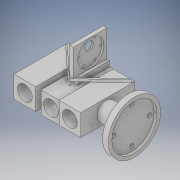
# Autodesk Inventor part: fingers1
Saved by Autodesk Inventor 2018 (Build 220112000, 112)
## iProperties
Created: 2020-03-06
Part Number: fingers1
Material: Generic
Document SubType Name: Modeling
Designer: Jesse R-B
Density: 1 g/cm^3
Appearance: Default
Author: Jesse R-B
Autodesk Inventor part; units mm, degrees
sketch "Sketch1" plane through (0, 0, 0) normal (1, 0, 0) x (0, 1, 0)
  circle A0 centre (0, 0) radius 2.9972
  dimension "d0" = 5.9944
  constraints: 1 centre point, 1 coincident
  measures "d0" diameter of A0
extrude "Extrusion1" add sketch "Sketch1" along normal blind 34.8234
sketch "Sketch2" plane through (34.8234, 0, 0) normal (1, 0, 0) x (0, 0, -1)
  circle A0 centre (0, 0) radius 15.24
  dimension "d3" = 30.48
  constraints: 1 centre point, 1 coincident
  measures "d3" diameter of A0
extrude "Extrusion2" add sketch "Sketch2" against normal blind 12.7
ref_plane "Work Plane1" through (0, 0, 0) normal (0, -0.8660254, 0.5) x (1, 0, 0)
sketch "Sketch7" plane through (0, 0, 0) normal (0, -0.8660254, 0.5) x (1, 0, 0)
  line L0 (34.8234, -9.1805) -> (22.1234, -9.1805) projected
  line L1 (22.1234, 6.4681) -> (22.1234, 5.3565) projected
  line L2 (34.8234, 6.4681) -> (22.1234, 6.4681) projected
  line L3 (34.8234, 6.4681) -> (34.8234, 5.3565) projected
  line L4 (22.1234, 4.8046) -> (34.8234, 4.8046)
  line L5 (34.8234, 4.8046) -> (34.8234, -7.8954)
  line L6 (34.8234, -7.8954) -> (22.1234, -7.8954)
  line L7 (22.1234, -7.8954) -> (22.1234, 4.8046)
  line L8 (22.1234, 2.9972) -> (22.1234, -2.9972) projected
  line L9 (0, 2.9972) -> (0, -2.9972) projected
  line L10 (0, 2.9972) -> (22.1234, 2.9972) projected
  line L11 (22.1234, 5.3565) -> (34.8234, 5.3565) projected
  point P0 (0, 0)
  dimension "d20" = 12.7
  constraints: 8 end point, 2 parallel, 1 horizontal, 1 perpendicular
  measures "d20" distance between parallel lines of L7 L5
extrude "Extrusion5" add sketch "Sketch7" along normal blind 38.1 contours L4 L5 L6 L7
sketch "Sketch8" plane through (34.8234, 0, 0) normal (1, 0, 0) x (0, 0, -1)
  line L0 (-11.3923, -10.1229) -> (-23.2109, -30.5933) projected
  line L1 (-23.2109, -30.5933) -> (-8.5462, -30.5933)
  line L2 (0.3199, -15.2366) -> (-12.2124, -36.9433) projected
  line L3 (-8.5462, -30.5933) -> (-12.2124, -36.9433)
  line L4 (-12.2124, -36.9433) -> (-23.2109, -30.5933)
  point P0 (0, 0)
  point P1 (0.1491, -15.5326)
  point P2 (-0.4582, -16.5843)
  point P3 (-11.957, -11.101)
  point P4 (0.2017, -15.4414)
  point P5 (-11.819, -10.8618)
  constraints: 6 end point, 1 collinear, 1 horizontal, 1 perpendicular, 1 point on line
extrude "Extrusion6" cut sketch "Sketch8" against normal blind 25.4
sketch "Sketch10" plane through (34.8234, -30.5933, 8.5462) normal (0, -1, 0) x (1, 0, 0)
  line L0 (-12.7, 0) -> (-12.7, 14.6647) projected
  line L1 (0, 0) -> (-12.7, 0) projected
  line L2 (0, 14.6647) -> (0, 0) projected
  line L3 (0, 14.6647) -> (-12.7, 14.6647) projected
  point P0 (-34.8234, -8.5462)
sketch "Sketch11" plane through (34.8234, -30.5933, 8.5462) normal (0, -1, 0) x (1, 0, 0)
  line L0 (7.62, 45.4323) -> (-20.32, 45.4323)
  line L1 (-20.32, 45.4323) -> (-20.32, -30.7677)
  line L2 (-20.32, -30.7677) -> (7.62, -30.7677)
  line L3 (7.62, -30.7677) -> (7.62, 45.4323)
  line L4 (0, 14.6647) -> (-12.7, 14.6647) construction
  line L5 (-6.35, 14.6647) -> (-6.35, 45.4323) construction
  line L6 (0, 0) -> (-12.7, 0) construction
  line L7 (-6.35, 0) -> (-6.35, -30.7677) construction
  line L8 (0, 2.8461) -> (0, 14.6647) construction
  line L9 (0, 8.9687) -> (7.62, 8.9687) construction
  line L10 (-12.7, 2.8461) -> (-12.7, 14.6647) construction
  line L11 (-12.7, 8.9687) -> (-20.32, 8.9687) construction
  point P0 (-34.8234, -8.5462)
  point P1 (0, 3.4108)
  point P2 (-12.7, 3.4108)
  point P3 (0, 3.2728)
  point P4 (-12.7, 3.2728)
  dimension "d29" = 27.94
  dimension "d30" = 76.2
  constraints: 16 end point, 6 point on line, 4 midpoint, 3 perpendicular, 2 collinear, 2 parallel, 1 horizontal
  measures "d29" distance between parallel lines of L3 L1
  measures "d30" distance of L2.end L0.start
extrude "Extrusion8" add sketch "Sketch11" along normal blind 30.48
sketch "Sketch13" plane through (14.5034, -30.5933, -22.2214) normal (-1, 0, 0) x (0, 0, 1)
  line L0 (45.6572, -16.7321) -> (32.9572, -16.7321)
  line L1 (32.9572, -16.7321) -> (32.9572, -4.0321)
  line L2 (32.9572, -4.0321) -> (45.6572, -4.0321)
  line L3 (45.6572, -4.0321) -> (45.6572, -16.7321)
  point P0 (22.2214, 30.5933)
  dimension "d37" = 12.7
  dimension "d38" = 12.7
  constraints: 8 end point, 2 parallel, 1 horizontal, 1 perpendicular
  measures "d37" distance of L0.start L0.end
  measures "d38" distance of L0.end L1.end
extrude "Extrusion9" add sketch "Sketch13" along normal blind 2.54
sketch "Sketch14" plane through (11.9634, -30.5933, -22.2214) normal (-1, 0, 0) x (0, 0, 1)
  line L0 (81.28, -25.4) -> (5.08, -25.4)
  line L1 (5.08, -25.4) -> (5.08, 5.08)
  line L2 (5.08, 5.08) -> (81.28, 5.08)
  line L3 (81.28, 5.08) -> (81.28, -25.4)
  line L4 (76.2, 0) -> (0, 0) projected
  line L5 (76.2, 0) -> (76.2, -30.48) projected
  point P0 (22.2214, 30.5933)
  dimension "d41" = 30.48
  dimension "d45" = 76.2
  dimension "d46" = 5.08
  dimension "d47" = 5.08
  constraints: 8 end point, 2 parallel, 1 horizontal, 1 perpendicular
  measures "d41" distance of L2.end L0.start
  measures "d45" distance of L1.end L2.end
  measures "d46" distance between parallel lines of L4 L2
  measures "d47" distance between parallel lines of L5 L3
extrude "Extrusion10" add sketch "Sketch14" along normal blind 30.48
ref_plane "Work Plane2" through (28.4734, -30.5933, -22.2214) normal (-1, 0, 0) x (0, 0, 1)
mirror "Mirror1" about plane through (28.4734, -30.5933, -22.2214) normal (-1, 0, 0) of "Extrusion10", "Extrusion9"
sketch "Sketch15" plane through (11.9634, -55.9933, -17.1414) normal (0, -1, 0) x (1, 0, 0)
  line L0 (33.02, 76.2) -> (33.02, 0) construction
  line L1 (33.02, 0) -> (63.5, 0) construction
  line L2 (63.5, 0) -> (63.5, 76.2) construction
  line L3 (33.02, 76.2) -> (63.5, 76.2) construction
  line L4 (30.48, 71.12) -> (2.54, 71.12) construction
  line L5 (2.54, 71.12) -> (2.54, -5.08) construction
  line L6 (2.54, -5.08) -> (30.48, -5.08) construction
  line L7 (30.48, -5.08) -> (30.48, 71.12) construction
  line L8 (0, 76.2) -> (0, 0) construction
  line L9 (0, 76.2) -> (-30.48, 76.2) construction
  line L10 (-30.48, 0) -> (-30.48, 76.2) construction
  line L11 (0, 0) -> (-30.48, 0) construction
  line L12 (33.02, 0) -> (63.5, 0) construction
  line L13 (63.5, 0) -> (16.7235, 43.4086) construction
  line L14 (0, 0) -> (-30.48, 0) construction
  line L15 (16.7235, 43.4086) -> (-30.48, 0) construction
  circle A0 centre (60.7629, 2.54) radius 2.54 construction
  line L16 (62.4907, 4.4018) -> (18.4513, 45.2705)
  line L17 (59.0352, 0.6782) -> (14.9957, 41.5468)
  arc A1 (59.0352, 0.6782) -> (62.4907, 4.4018) centre (60.7629, 2.54) ccw
  arc A2 (18.4513, 45.2705) -> (14.9957, 41.5468) centre (16.7235, 43.4086) ccw
  point P0 (-11.9634, 17.1414)
  dimension "d50" = 5.08
  dimension "d52" = 5.08
  constraints: 8 end point, 6 point on circle, 3 centre point, 3 tangent, 1 coincident, 1 concentric, 1 parallel, 1 point on line
  measures "d50" diameter of A0
  measures "d52" diameter of A2
extrude "Extrusion11" add sketch "Sketch15" along normal blind 2.54 draft -30
mirror "Mirror2" about plane through (28.4734, -30.5933, -22.2214) normal (-1, 0, 0) of "Extrusion11"
sketch "Sketch16" plane through (14.5034, -30.5933, 53.9786) normal (0, 0, 1) x (1, 0, 0)
  line L0 (27.94, 0) -> (0, 0) projected
  line L1 (0, 0) -> (0, -30.48) projected
  line L2 (27.94, -30.48) -> (0, -30.48) projected
  line L3 (27.94, 0) -> (27.94, -30.48) projected
  circle A0 centre (13.97, -15.24) radius 10.541
  line L4 (30.48, 5.08) -> (30.48, -25.4) projected
  line L5 (30.48, -25.4) -> (60.96, -25.4) projected
  line L6 (60.96, -25.4) -> (60.96, 5.08) projected
  line L7 (30.48, 5.08) -> (60.96, 5.08) projected
  line L8 (-2.54, 5.08) -> (-2.54, -25.4) projected
  line L9 (-2.54, 5.08) -> (-33.02, 5.08) projected
  line L10 (-33.02, -25.4) -> (-33.02, 5.08) projected
  line L11 (-2.54, -25.4) -> (-33.02, -25.4) projected
  circle A1 centre (45.72, -10.16) radius 10.541
  circle A2 centre (-17.78, -10.16) radius 10.541
  point P0 (-14.5034, 30.5933)
  dimension "d56" = 21.082
  dimension "d57" = 21.082
  dimension "d58" = 15.24
  dimension "d59" = 15.24
  dimension "d62" = 15.24
  dimension "d63" = 15.24
  dimension "d64" = 21.082
  dimension "d66" = 13.97
  dimension "d67" = 15.24
  constraints: 3 centre point
  measures "d56" diameter of A1
  measures "d57" diameter of A2
  measures "d58" distance from line of L5 A1.centre
  measures "d59" distance from line of L6 A1.centre
  measures "d62" distance from line of L11 A2.centre
  measures "d63" distance from line of L10 A2.centre
  measures "d64" diameter of A0
  measures "d66" distance from line of L3 A0.centre
  measures "d67" distance from line of L2 A0.centre
extrude "Extrusion12" cut sketch "Sketch16" along normal through all both and the other way through all contours A0 | A1 | A2
ref_plane "Work Plane3" through (-18.5166, -40.7533, 59.0586) normal (0, -1, 0) x (1, 0, 0)
mirror "Mirror3" about plane through (-18.5166, -40.7533, 59.0586) normal (0, -1, 0) of "Extrusion11", "Mirror2"
sketch "Sketch17" plane through (31.4068, -25.5133, 20.278) normal (0, -1, 0) x (1, 0, 0)
  line L0 (-46.456, -35.6663) -> (-2.9334, 4.7228) projected
  arc A0 (-47.9165, -34.0925) -> (-46.456, -35.6663) centre (-47.1863, -34.8794) ccw projected
  line L1 (-3.8771, 6.7761) -> (-47.9165, -34.0925) projected
  arc A1 (-2.9334, 7.0413) -> (-3.8771, 6.7761) centre (-3.1468, 5.9892) ccw projected
  arc A2 (-1.9896, 6.7761) -> (-2.9334, 7.0413) centre (-2.7199, 5.9892) ccw projected
  line L2 (-1.9896, 6.7761) -> (42.0498, -34.0925) projected
  arc A3 (40.5893, -35.6663) -> (42.0498, -34.0925) centre (41.3196, -34.8794) ccw projected
  line L3 (40.5893, -35.6663) -> (-2.9334, 4.7228) projected
  line L4 (-2.9334, 7.0413) -> (-2.9334, 8.5202) projected
  arc A4 (-2.9334, 7.0413) -> (-3.8771, 6.7761) centre (-3.1468, 5.9892) ccw projected
  line L5 (-4.8746, 7.8511) -> (-3.8771, 6.7761) projected
  arc A5 (-2.9334, 8.5202) -> (-4.8746, 7.8511) centre (-3.1468, 5.9892) ccw projected
  line L6 (-2.9334, 7.0413) -> (-2.9334, 8.5202) projected
  arc A6 (-0.9921, 7.8511) -> (-2.9334, 8.5202) centre (-2.7199, 5.9892) ccw projected
  line L7 (-0.9921, 7.8511) -> (-1.9896, 6.7761) projected
  arc A7 (-1.9896, 6.7761) -> (-2.9334, 7.0413) centre (-2.7199, 5.9892) ccw projected
  circle A8 centre (-2.9334, 7.0413) radius 1.4789
  point P0 (-31.4068, -20.278)
  constraints: 1 coincident, 1 vertical alignment, 2 other
extrude "Extrusion13" add sketch "Sketch17" along normal blind 7.62 contours A8 L5 L1 | L1 A1 A2 L2 A8 | L5 A8 L4 A1 | L2 L7 A8 | L4 A8 L7 A2
ref_plane "Work Plane4" through (15.7734, 0, 0) normal (-1, 0, 0) x (0, 0, 1)
sketch "Sketch19" plane through (34.8234, 0, 0) normal (1, 0, 0) x (0, 0, -1)
  line L0 (-27.0541, -22.9733) -> (13.8145, -22.9733) projected
  line L1 (-49.0455, 45.2859) -> (19.1397, 45.2859)
  line L2 (19.1397, 45.2859) -> (19.1397, -22.9733)
  line L3 (19.1397, -22.9733) -> (-49.0455, -22.9733)
  line L4 (-49.0455, -22.9733) -> (-49.0455, 45.2859)
  point P0 (0, 0)
  constraints: 8 end point, 2 parallel, 1 horizontal, 1 perpendicular
extrude "Extrusion15" cut sketch "Sketch19" against normal blind 76.2
sketch "Sketch20" plane through (34.8234, -22.9733, 18.8115) normal (0, 1, 0) x (1, 0, 0)
  line L0 (-12.7, 14.6647) -> (0, 14.6647) projected
  line L1 (-12.7, 0) -> (-12.7, 14.6647) projected
  line L2 (0, 0) -> (-12.7, 0) projected
  line L3 (0, 14.6647) -> (0, 0) projected
  line L4 (39.6307, 31.5511) -> (10.16, 4.2023) projected
  line L5 (10.16, 4.2023) -> (10.16, -40.2471) projected
  line L6 (10.16, -40.2471) -> (40.64, -40.2471) projected
  line L7 (40.64, -40.2471) -> (40.64, 35.9529) projected
  line L8 (37.9029, 35.9529) -> (40.64, 35.9529) projected
  arc A0 (39.6307, 31.5511) -> (37.9029, 35.9529) centre (37.9029, 33.4129) ccw projected
  arc A1 (-50.6029, 35.9529) -> (-52.3307, 31.5511) centre (-50.6029, 33.4129) ccw projected
  line L9 (-50.6029, 35.9529) -> (-53.34, 35.9529) projected
  line L10 (-53.34, -40.2471) -> (-53.34, 35.9529) projected
  line L11 (-22.86, -40.2471) -> (-53.34, -40.2471) projected
  line L12 (-22.86, 4.2023) -> (-22.86, -40.2471) projected
  line L13 (-22.86, 4.2023) -> (-52.3307, 31.5511) projected
  line L14 (-12.7, 0) -> (-12.7, 14.6647) projected
  line L15 (-12.7, 7.3323) -> (0, 7.3323)
  line L16 (0, 7.3323) -> (0, 39.0823)
  line L17 (0, 39.0823) -> (-12.7, 39.0823)
  line L18 (-12.7, 39.0823) -> (-12.7, 7.3323)
  point P0 (-34.8234, 18.8115)
  dimension "d78" = 31.75
  dimension "d79" = 0
  constraints: 8 end point, 2 parallel, 1 horizontal, 1 midpoint, 1 perpendicular
  measures "d78" distance of L17.end L15.start
  measures "d79" distance between parallel lines of L3 L16
extrude "Extrusion16" add sketch "Sketch20" against normal up to surface (7.62 mm away) contours L18 L17 L16 L0 | L0 L3 L15 L1 | L15 L3 L2 L1
ref_plane "Work Plane5" through (28.4734, 0, 0) normal (1, 0, 0) x (0, 0, -1)
sketch "Sketch21" plane through (28.4734, 0, 0) normal (1, 0, 0) x (0, 0, -1)
  circle A0 centre (-0.349, 3.0767) radius 5.9944
  circle A1 centre (15.151, -3.9233) radius 1.4986
  circle A2 centre (7.401, 9.5001) radius 1.4986
  circle A3 centre (-8.099, 9.5001) radius 1.4986
  circle A4 centre (-15.849, -3.9233) radius 1.4986
  circle A5 centre (-8.099, -17.3467) radius 1.4986
  circle A6 centre (7.401, -17.3467) radius 1.4986
  circle A7 centre (-0.349, -3.9233) radius 18.4023
  circle A8 centre (-0.349, -3.9233) radius 18.4023
  line L0 (18.193, 15.1267) -> (15.3215, 15.1267)
  line L1 (-16.0195, 15.1267) -> (15.3215, 15.1267)
  line L2 (-16.0195, 15.1267) -> (-18.891, 15.1267)
  line L3 (-18.891, 15.1267) -> (-18.891, -22.9733)
  line L4 (-16.0195, -22.9733) -> (-18.891, -22.9733)
  line L5 (15.3215, -22.9733) -> (-16.0195, -22.9733)
  line L6 (18.193, -22.9733) -> (15.3215, -22.9733)
  line L7 (18.193, 15.1267) -> (18.193, -22.9733)
  line L8 (-16.0195, 15.1267) -> (15.3215, 15.1267)
  line L9 (-27.0541, -22.9733) -> (13.8145, -22.9733) projected
  line L10 (20.2708, -22.9733) -> (20.2708, -30.5933) projected
  point P0 (0, 0)
  dimension "d82" = 36.8046
  dimension "d83" = 11.9888
  dimension "d84" = 2.9972
  dimension "d85" = 2.9972
  dimension "d86" = 2.9972
  dimension "d87" = 2.9972
  dimension "d88" = 2.9972
  dimension "d89" = 2.9972
  dimension "d90" = 90
  dimension "d91" = 2.8715
  dimension "d92" = 31.341
  dimension "d93" = 31.341
  dimension "d94" = 38.1
  dimension "d95" = 37.084
  dimension "d96" = 7
  dimension "d97" = 18.542
  dimension "d98" = 18.542
  dimension "d99" = 7
  dimension "d100" = 19.05
  dimension "d101" = 6.4234
  dimension "d102" = 7.75
  dimension "d103" = 6.4234
  dimension "d104" = 7.75
  dimension "d105" = 15.5
  dimension "d106" = 9.5144
  dimension "d107" = 15.5
  dimension "d108" = 7
  dimension "d109" = 13.4234
  dimension "d110" = 7.75
  dimension "d111" = 7.75
  dimension "d112" = 20.4234
  dimension "d113" = 0
  dimension "d114" = 2.0778
  dimension "d115" = 15.1267
  constraints: 18 end point, 9 centre point, 2 collinear, 2 concentric
  measures "d82" diameter of A7
  measures "d83" diameter of A0
  measures "d84" diameter of A3
  measures "d85" diameter of A2
  measures "d86" diameter of A1
  measures "d87" diameter of A6
  measures "d88" diameter of A5
  measures "d89" diameter of A4
  measures "d90" angle of L1 L3
  measures "d91" distance from line of L7 L1.end
  measures "d92" distance of L1.start L1.end
  measures "d93" distance of L5.start L4.start
  measures "d94" distance of L0.start L7.end
  measures "d95" distance between parallel lines of L3 L7
  measures "d96" distance of A8.centre A0.centre
  measures "d97" distance from line of L7 A8.centre
  measures "d98" distance from line of L3 A0.centre
  measures "d99" distance of A7.centre A0.centre
  measures "d100" distance from line of A8.centre L5
  measures "d101" vertical distance of A0.centre A2.centre
  measures "d102" horizontal distance of A0.centre A2.centre
  measures "d103" vertical distance of A3.centre A0.centre
  measures "d104" horizontal distance of A3.centre A0.centre
  measures "d105" horizontal distance of A0.centre A4.centre
  measures "d107" horizontal distance of A0.centre A1.centre
  measures "d108" vertical distance of A0.centre A1.centre
  measures "d109" vertical distance of A6.centre A1.centre
  measures "d110" horizontal distance of A1.centre A6.centre
  measures "d111" horizontal distance of A0.centre A5.centre
  measures "d112" vertical distance of A0.centre A5.centre
  measures "d113" distance between parallel lines of L9 L5
  measures "d114" distance between parallel lines of L10 L7
  measures "d115" distance from line of point (0, 0) L1
extrude "Extrusion17" add sketch "Sketch21" along normal mid plane 5.08 contours L7 L6 L5 L4 L3 L2 L1 L0
extrude "Extrusion18" add sketch "Sketch21" against normal blind 2.54 contours A7
sketch "Sketch22" plane through (34.8234, -22.9733, -20.2708) normal (0, 0, -1) x (-1, 0, 0)
  line L0 (6.35, 0.6477) -> (6.35, 37.4523) projected
  line L1 (8.89, 38.1) -> (3.81, 38.1) projected
  line L2 (3.81, 0) -> (3.81, 38.1) projected
  line L3 (8.89, 0) -> (3.81, 0) projected
  line L4 (8.89, 38.1) -> (8.89, 0) projected
  line L5 (12.7, -7.62) -> (0, -7.62) projected
  line L6 (12.7, 0) -> (12.7, -7.62) projected
  line L7 (0, 0) -> (12.7, 0) projected
  line L8 (0, 0) -> (0, -7.62) projected
  point P0 (34.8234, 22.9733)
extrude "Extrusion19" add sketch "Sketch22" against normal up to surface (2.0778 mm away) contours L4 L3 L2 L1
sketch "Sketch23" plane through (34.8234, -30.5933, -20.2708) normal (0, 0, -1) x (-1, 0, 0)
  line L0 (12.7, 0) -> (0, 0) projected
  line L1 (12.7, 7.62) -> (12.7, 0) projected
  line L2 (8.89, 7.62) -> (12.7, 7.62) projected
  line L3 (8.89, 7.62) -> (8.89, 45.72) projected
  line L4 (8.89, 45.72) -> (3.81, 45.72) projected
  line L5 (3.81, 45.72) -> (3.81, 7.62) projected
  line L6 (0, 7.62) -> (3.81, 7.62) projected
  line L7 (0, 7.62) -> (0, 0) projected
  point P0 (34.8234, 30.5933)
extrude "Extrusion20" add sketch "Sketch23" along normal up to surface (1.9506 mm away)
sketch "Sketch29" plane through (25.9334, -22.9733, 18.891) normal (0, 0, 1) x (1, 0, 0)
  line L0 (2.54, 37.4523) -> (2.54, 0.6477) projected
  line L1 (0, 0) -> (5.08, 0) projected
  line L2 (5.08, 38.1) -> (5.08, 0) projected
  line L3 (0, 38.1) -> (5.08, 38.1) projected
  line L4 (0, 0) -> (0, 38.1) projected
  point P0 (-25.9334, 22.9733)
extrude "Extrusion23" add sketch "Sketch29" along normal blind 6.35
sketch "Sketch30" plane through (75.4634, -55.9933, -17.1414) normal (1, 0, 0) x (0, 0, -1)
  line L0 (0, 0) -> (-76.2, 0) projected
  line L1 (0, 30.48) -> (0, 0) projected
  line L2 (-76.2, 30.48) -> (0, 30.48) projected
  line L3 (-76.2, 0) -> (-76.2, 30.48) projected
  line L4 (-40.5772, 8.6679) -> (-40.5772, 21.3679) projected
  circle A0 centre (-40.5772, 15.0179) radius 12.7
  point P0 (-17.1414, 55.9933)
  dimension "d132" = 25.4
  constraints: 1 centre point, 1 midpoint
  measures "d132" diameter of A0
extrude "Extrusion24" add sketch "Sketch30" along normal blind 31.9532 contours A0
sketch "Sketch31" plane through (107.4166, -40.9754, 23.4357) normal (1, 0, 0) x (0, 0, -1)
  circle A0 centre (0, 25) radius 2.921
  circle A1 centre (25, 0) radius 2.921
  circle A2 centre (0, -25) radius 2.921
  circle A3 centre (-25, 0) radius 2.921
  circle A4 centre (0, 0) radius 31.75
  circle A5 centre (0, 0) radius 31.75
  circle A6 centre (0, 0) radius 36.83
  point P0 (23.4357, 40.9754)
  dimension "d135" = 5.842
  dimension "d136" = 73.66
  dimension "d137" = 63.5
  dimension "d138" = 63.5
  dimension "d139" = 41.0053
  dimension "d140" = 28.3628
  dimension "d141" = 47.204
  dimension "d142" = 47.204
  dimension "d143" = 70.0142
  dimension "d144" = 63.4429
  dimension "d145" = 47.204
  dimension "d146" = 35.3553
  dimension "d147" = 25
  dimension "d148" = 25
  dimension "d149" = 25
  dimension "d150" = 35.3553
  dimension "d151" = 50
  constraints: 7 centre point, 3 equal radius, 1 concentric
  measures "d135" diameter of A1
  measures "d136" diameter of A6
  measures "d137" diameter of A4
  measures "d138" diameter of A5
  measures "d139" distance of point (23.436, 40.975) A1.centre
  measures "d140" distance of point (23.436, 40.975) A0.centre
  measures "d141" distance of point (23.436, 40.975) A4.centre
  measures "d142" distance of point (23.436, 40.975) point (0, 0)
  measures "d143" distance of point (23.436, 40.975) A2.centre
  measures "d144" distance of point (23.436, 40.975) A3.centre
  measures "d145" distance of A5.centre point (23.436, 40.975)
  measures "d146" distance of A1.centre A0.centre
  measures "d147" distance of A1.centre A4.centre
  measures "d148" distance of A5.centre A1.centre
  measures "d149" distance of point (0, 0) A1.centre
  measures "d150" distance of A1.centre A2.centre
  measures "d151" distance of A1.centre A3.centre
extrude "Extrusion25" add sketch "Sketch31" along normal blind 3.9878 contours A4 | A6
extrude "Extrusion26" add sketch "Sketch31" along normal blind 8.0518 contours A6
body "Solid1"
